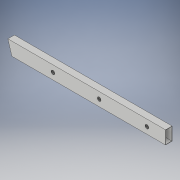
# Autodesk Inventor part: Aluminum Channel Arm Left
Saved by Autodesk Inventor 2019 (Build 230136000, 136)
## iProperties
Created: 2019-01-26
Part Number: Aluminum Channel Arm Left
Material: Generic
Document SubType Name: Modeling
Designer: josh
Density: 1 g/cm^3
Appearance: Default
Author: josh
Autodesk Inventor part; units mm, degrees
ref_plane "YZ Plane" through (0, 0, 0) normal (1, 0, 0) x (0, 1, 0)
ref_plane "XZ Plane" through (0, 0, 0) normal (0, 1, 0) x (-1, 0, 0)
ref_plane "XY Plane" through (0, 0, 0) normal (0, 0, 1) x (1, 0, 0)
sketch "Sketch1" plane through (0, 0, 0) normal (1, 0, 0) x (0, 1, 0)
  line L0 (0, 0) -> (50.8, 0)
  line L1 (50.8, 0) -> (50.8, -25.4)
  line L2 (50.8, -25.4) -> (0, -25.4)
  line L3 (0, -25.4) -> (0, 0)
  line L4 (49.53, -24.13) -> (49.53, -1.27)
  line L5 (49.53, -1.27) -> (1.27, -1.27)
  line L6 (1.27, -1.27) -> (1.27, -24.13)
  line L7 (1.27, -24.13) -> (49.53, -24.13)
  dimension "d0" = 50.8
  dimension "d1" = 25.4
  dimension "d2" = 1.27
  constraints: 16 end point, 4 parallel, 2 perpendicular, 1 horizontal, 3 other
  measures "d0" distance of L1.end L2.end
  measures "d1" distance of L0.end L1.end
  measures "d2" distance between parallel lines of L1 L4
extrude "Extrusion1" add sketch "Sketch1" along normal blind 609.6
sketch "Sketch2" plane through (0, 0, 0) normal (0, 0, 1) x (1, 0, 0)
  line L0 (537.5598, 19.0095) -> (541.0559, 18.8772) projected
  line L1 (534.0637, 19.1419) -> (537.5598, 19.0095) projected
  line L2 (532.1846, 22.3903) -> (533.818, 19.2964) projected
  arc A0 (533.818, 19.2964) -> (534.0637, 19.1419) centre (537.8, 25.355) ccw projected
  arc A1 (530.5621, 25.7742) -> (530.5512, 25.4841) centre (537.8, 25.355) ccw projected
  arc A2 (534.5441, 31.8328) -> (534.2874, 31.6973) centre (537.8, 25.355) ccw projected
  arc A3 (541.782, 31.4136) -> (541.5363, 31.5681) centre (537.8, 25.355) ccw projected
  arc A4 (545.0379, 24.9358) -> (545.0488, 25.2259) centre (537.8, 25.355) ccw projected
  arc A5 (541.0559, 18.8772) -> (541.3126, 19.0127) centre (537.8, 25.355) ccw projected
  circle A6 centre (537.8, 25.355) radius 7.25
  point P0 (0, 0)
  constraints: 1 coincident, 3 other
extrude "Extrusion2" cut sketch "Sketch2" against normal through all
sketch "Sketch4" plane through (0, 0, 0) normal (0, 0, 1) x (1, 0, 0)
  circle A0 centre (352.9118, 25.4) radius 7.3323
  circle A1 centre (174.2245, 25.4) radius 7.3323
  point P0 (0, 0)
  constraints: 2 centre point
extrude "Extrusion4" cut sketch "Sketch4" against normal through all
sketch "Sketch5" plane through (0, 0, -25.4) normal (0, 0, -1) x (-1, 0, 0)
  line L0 (0, 50.8) -> (-609.6, 50.8) projected
  line L1 (0, 50.8) -> (-15.2407, 0)
  line L2 (0, 0) -> (-609.6, 0) projected
  line L3 (0, 50.8) -> (53.037, 50.8) construction
  line L4 (0, 50.8) -> (0, 0)
  line L5 (0, 0) -> (-15.2407, 0)
  line L6 (0, 1.27) -> (-609.6, 1.27) projected
  dimension "d12" = 106.7
  constraints: 8 end point, 1 equal length, 1 horizontal, 1 parallel, 1 point on line, 1 vertical
  measures "d12" angle of L1 L3
extrude "Extrusion5" cut sketch "Sketch5" against normal blind 25.4
body "Solid1"
